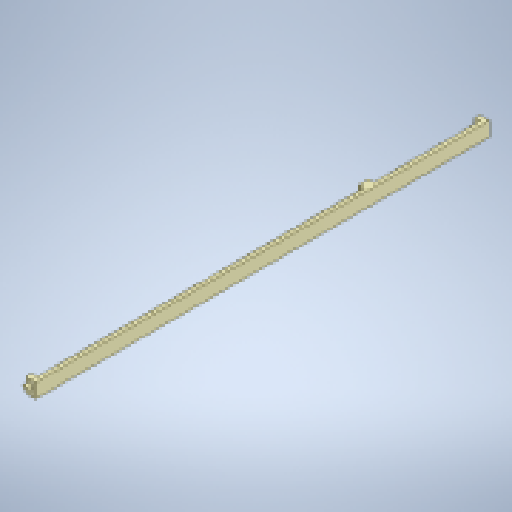
# Autodesk Inventor part: Case Rail
Saved by Autodesk Inventor 2025 (Build 290162000, 162)
## iProperties
Created: 2024-07-16
Part Number: Case Rail
Material: PET Plastic
Document SubType Name: Modeling
Designer: adam
Density: 1.541 g/cm^3
Appearance: Smooth - Ash
Author: adam
Autodesk Inventor part; units mm, degrees
ref_plane "YZ Plane" through (0, 0, 0) normal (1, 0, 0) x (0, 1, 0)
ref_plane "XZ Plane" through (0, 0, 0) normal (0, 1, 0) x (-1, 0, 0)
ref_plane "XY Plane" through (0, 0, 0) normal (0, 0, 1) x (1, 0, 0)
sketch "Sketch1" plane through (0, 0, 0) normal (0, 0, 1) x (1, 0, 0)
  line L0 (0, 3.75) -> (2, 3.75)
  line L1 (2, 3.75) -> (2, -4)
  line L2 (2, -4) -> (0, -4)
  line L3 (0, -4) -> (0, 3.75) construction
  line L4 (0, -4) -> (-5, -4)
  line L5 (-5, -4) -> (-5, -1)
  line L6 (-5, -1) -> (0, -1)
  line L7 (0, 3.75) -> (-1, 3.75)
  line L8 (-1, 3.75) -> (-1, 0.75)
  line L9 (-1, 0.75) -> (0, 0.75)
  line L10 (0, 0.75) -> (0, 3.75) construction
  line L11 (0, 0.75) -> (0, -1)
  point P0 (0, 0)
  point P1 (0, -0.125)
  point P2 (1, 3.75)
  dimension "d0" = 4
  dimension "d1" = 2
  dimension "d5" = 5
  dimension "d6" = 1.75
  dimension "d7" = 3
  dimension "d11" = 3
  dimension "d12" = 3
  constraints: 24 end point, 5 parallel, 3 horizontal, 3 perpendicular, 2 midpoint, 1 collinear, 1 point on line
  measures "d0" distance from line of L2 point (0, 0)
  measures "d1" distance from line of L1 point (0, -0.125)
  measures "d5" distance between parallel lines of L3 L5
  measures "d6" distance between parallel lines of L6 L9
  measures "d7" distance of L4.end L5.end
  measures "d11" distance between parallel lines of L0 L9
  measures "d12" distance between parallel lines of L1 L8
extrude "Extrusion1" add sketch "Sketch1" along normal blind 243.25
sketch "Sketch2" plane through (-1, 0.75, 0) normal (-1, 0, 0) x (0, 0, 1)
  line L0 (0, 3) -> (0, 0) projected
  line L1 (0, 0) -> (243.25, 0) projected
  line L2 (243.25, 3) -> (243.25, 0) projected
  line L3 (0, 3) -> (243.25, 3) projected
  point P0 (0, -0.75)
extrude "Extrusion2" cut sketch "Sketch2" against normal blind 0.9
chamfer "Chamfer1" distance 2.5 angle 45 1 edges at (-5, -4, 121.625)
sketch "Sketch3" plane through (-0.1, 0.75, 0) normal (-1, 0, 0) x (0, 0, 1)
  line L0 (0, 3) -> (243.25, 3) projected
  line L1 (0, 3) -> (2.95, 3)
  line L2 (2.95, 3) -> (2.95, 0.55)
  line L3 (2.95, 0.55) -> (0, 0.55)
  line L4 (0, 0.55) -> (0, 3)
  line L5 (59.8466, 2.85) -> (59.8466, 0.85) construction
  line L6 (59.8466, 2.85) -> (59.8466, 3) construction
  line L7 (59.8466, 3) -> (64.7966, 3)
  line L8 (64.7966, 3) -> (64.7966, 0.55)
  line L9 (64.7966, 0.55) -> (59.8466, 0.55)
  line L10 (59.8466, 0.55) -> (59.8466, 3)
  line L11 (243.25, 3) -> (243.25, 0) projected
  line L12 (243.25, 3) -> (240.3, 3)
  line L13 (240.3, 3) -> (240.3, 0.55)
  line L14 (240.3, 0.55) -> (243.25, 0.55)
  line L15 (243.25, 0.55) -> (243.25, 3)
  point P0 (0, -0.75)
  dimension "d18" = 2.45
  dimension "d19" = 2.95
  dimension "d20" = 4.95
  dimension "d21" = 2.45
  dimension "d22" = 2.45
  dimension "d23" = 2.95
  constraints: 26 end point, 6 parallel, 4 perpendicular, 3 horizontal, 1 point on line
  measures "d18" distance of L1.end L2.end
  measures "d19" distance of L2.end L3.end
  measures "d20" distance of L8.end L9.end
  measures "d21" distance of L9.end L6.end
  measures "d22" distance of L12.end L13.end
  measures "d23" distance of L13.end L14.end
extrude "Extrusion3" add sketch "Sketch3" along normal blind 2.95
sketch "Sketch4" plane through (2, -4, 0) normal (0, -1, 0) x (1, 0, 0)
  circle A0 centre (-4.4525, -10.6025) radius 0.725 construction
  line L0 (-3.2, -15.005) -> (-3.2, -1) construction
  line L1 (-4.5, 0) -> (0, 0) construction
  line L2 (-4.5, 243.25) -> (0, 243.25) construction
  circle A1 centre (-10.2025, 230.7475) radius 2.55 construction
  circle A2 centre (-10.1275, 141.3958) radius 2.55 construction
  circle A3 centre (-10.2025, 51.9975) radius 2.55 construction
  circle A4 centre (-10.2025, 29.9975) radius 2.55 construction
  circle A5 centre (-10.2025, 10.9975) radius 2.55 construction
  line L3 (-3.2, 6.8975) -> (-7, 6.8975)
  line L4 (-7, 6.8975) -> (-7, 16.8975)
  line L5 (-7, 16.8975) -> (-3.2, 16.8975)
  line L6 (-3.2, 16.8975) -> (-3.2, 6.8975)
  line L7 (-3.2, 25.8975) -> (-7, 25.8975)
  line L8 (-7, 25.8975) -> (-7, 35.8975)
  line L9 (-7, 35.8975) -> (-3.2, 35.8975)
  line L10 (-3.2, 35.8975) -> (-3.2, 25.8975)
  line L11 (-3.2, 47.8975) -> (-7, 47.8975)
  line L12 (-7, 47.8975) -> (-7, 57.8975)
  line L13 (-7, 57.8975) -> (-3.2, 57.8975)
  line L14 (-3.2, 57.8975) -> (-3.2, 47.8975)
  line L15 (-3.2, 137.2957) -> (-7, 137.2957)
  line L16 (-7, 137.2957) -> (-7, 147.2957)
  line L17 (-7, 147.2957) -> (-3.2, 147.2957)
  line L18 (-3.2, 147.2957) -> (-3.2, 137.2957)
  line L19 (-2.1, 243.25) -> (-2.1, 0) projected
  line L20 (-2.1, 236.6475) -> (-2.1, 226.6475)
  circle A6 centre (-10.2025, -8.0025) radius 2.55 construction
  circle A7 centre (-5.5025, -3.6025) radius 0.725 construction
  line L21 (-3.2, -12.1025) -> (-10.2025, -12.1025) construction
  line L22 (-10.2025, -12.1025) -> (-10.2025, -2.1025) construction
  line L23 (-10.2025, -2.1025) -> (-3.2, -2.1025) construction
  line L24 (-7, 243.25) -> (-7, 0) construction
  line L25 (-7, 0) -> (-7, 243.25) projected
  line L26 (-7, 226.6475) -> (-3.2, 226.6475)
  line L27 (-3.2, 226.6475) -> (-3.2, 236.6475)
  line L28 (-3.2, 236.6475) -> (-7, 236.6475)
  line L29 (-7, 236.6475) -> (-7, 226.6475)
  point P0 (-2, 0)
  dimension "d26" = 1.5
  dimension "d27" = 1.5
  dimension "d28" = 4.1
  dimension "d29" = 5.9
  dimension "d30" = 4.1
  dimension "d31" = 5.9
  dimension "d32" = 4.1
  dimension "d33" = 5.9
  dimension "d34" = 4.1
  dimension "d35" = 5.9
  dimension "d36" = 4.1
  dimension "d37" = 5.9
  dimension "d40" = 4.1
  dimension "d41" = 5.9
  constraints: 48 end point, 10 parallel, 8 perpendicular, 7 collinear, 6 point on line, 5 horizontal, 2 other
  measures "d26" distance from line of L21 A0.centre
  measures "d27" distance from line of L23 A7.centre
  measures "d28" distance from line of A6.centre L21
  measures "d29" distance from line of L23 A6.centre
  measures "d30" distance from line of A5.centre L3
  measures "d31" distance from line of L5 A5.centre
  measures "d32" distance from line of A4.centre L7
  measures "d33" distance from line of L9 A4.centre
  measures "d34" distance from line of L11 A3.centre
  measures "d35" distance from line of L13 A3.centre
  measures "d36" distance from line of A2.centre L15
  measures "d37" distance from line of L17 A2.centre
  measures "d40" distance from line of A1.centre L26
  measures "d41" distance from line of A1.centre L28
extrude "Extrusion4" cut sketch "Sketch4" against normal up to surface (3 mm away)
equation "\"d21\" = d18"
equation "\"d22\" = d18"
equation "\"d30\" = d28"
equation "\"d31\" = d29"
equation "\"d32\" = d28"
equation "\"d33\" = d29"
equation "\"d34\" = d28"
equation "\"d35\" = d29"
equation "\"d36\" = d28"
equation "\"d37\" = d29"
equation "\"d40\" = d28"
equation "\"d41\" = d29"
body "Solid1"
